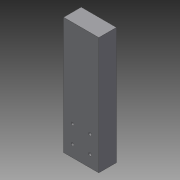
# Autodesk Inventor part: Arm-SquareBar-Rev3
Saved by Autodesk Inventor 2015 (Build 190159000, 159)
## iProperties
Created: 2017-01-08
Part Number: Arm-SquareBar-Rev3
Material: Generic
Document SubType Name: Modeling
Designer: Guy
Density: 1 g/cm^3
Appearance: Default
Author: Guy
Autodesk Inventor part; units mm, degrees
ref_plane "YZ Plane" through (0, 0, 0) normal (1, 0, 0) x (0, 1, 0)
ref_plane "XZ Plane" through (0, 0, 0) normal (0, 1, 0) x (-1, 0, 0)
ref_plane "XY Plane" through (0, 0, 0) normal (0, 0, 1) x (1, 0, 0)
sketch "Sketch1" plane through (0, 0, 0) normal (0, 0, 1) x (1, 0, 0)
  line L0 (0, 0) -> (60, 0)
  line L1 (60, 0) -> (60, 20)
  line L2 (60, 20) -> (0, 20)
  line L3 (0, 20) -> (0, 0)
  dimension "d0" = 60
  dimension "d1" = 20
  constraints: 8 end point, 2 parallel, 1 horizontal, 1 perpendicular
  measures "d0" distance of L1.end L2.end
  measures "d1" distance of L0.end L1.end
extrude "Extrusion1" add sketch "Sketch1" along normal blind 200
sketch "Sketch2" plane through (0, 0, 0) normal (0, -1, 0) x (1, 0, 0)
  line L0 (0, 0) -> (60, 0) projected
  line L1 (60, 0) -> (60, 200) projected
  line L2 (0, 200) -> (60, 200) projected
  line L3 (0, 0) -> (0, 200) projected
  circle A0 centre (15, 20) radius 2.5
  circle A1 centre (45, 20) radius 2.5
  circle A2 centre (15, 50) radius 2.5
  circle A3 centre (45, 50) radius 2.5
  dimension "d4" = 30
  dimension "d5" = 5
  dimension "d6" = 5
  dimension "d7" = 15
  dimension "d8" = 30
  dimension "d9" = 15
  dimension "d10" = 5
  dimension "d11" = 5
  dimension "d12" = 20
  dimension "d13" = 20
  dimension "d14" = 30
  dimension "d15" = 30
  constraints: 4 centre point
  measures "d4" distance of A3.centre A2.centre
  measures "d5" diameter of A2
  measures "d6" diameter of A3
  measures "d7" distance from line of L3 A2.centre
  measures "d8" distance of A1.centre A0.centre
  measures "d9" distance from line of L3 A0.centre
  measures "d10" diameter of A0
  measures "d11" diameter of A1
  measures "d12" distance from line of L0 A1.centre
  measures "d13" distance from line of L0 A0.centre
  measures "d14" distance of A2.centre A0.centre
  measures "d15" distance of A1.centre A3.centre
extrude "Extrusion2" cut sketch "Sketch2" against normal blind 200 contours A0 | A1 | A2 | A3
sketch "Sketch3" plane through (0, 0, 0) normal (-1, 0, 0) x (0, 0, 1)
  line L0 (0, 20) -> (0, 0) projected
  line L1 (0, 0) -> (200, 0) projected
  line L2 (200, 20) -> (200, 0) projected
  line L3 (0, 20) -> (200, 20) projected
  circle A0 centre (190, 10) radius 2.5
  circle A1 centre (180, 10) radius 2.5
  dimension "d18" = 5
  dimension "d19" = 5
  dimension "d22" = 10
  dimension "d24" = 10
  dimension "d26" = 10
  dimension "d27" = 10
  constraints: 2 centre point
  measures "d18" diameter of A0
  measures "d19" diameter of A1
  measures "d22" distance from line of L3 A0.centre
  measures "d24" distance from line of L3 A1.centre
  measures "d26" distance from line of L2 A0.centre
  measures "d27" distance of A1.centre A0.centre
extrude "Extrusion3" cut sketch "Sketch3" against normal through all contours A0 | A1
body "Solid1"
